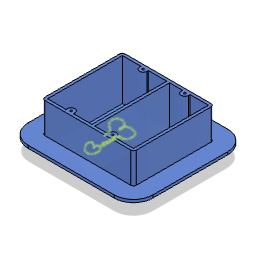
two-gang thicc (Autodesk Fusion 360 design; units mm, degrees)
Autodesk Fusion 360 part; units mm, degrees
note: some values were not read from the file. Set by a fixed rule: which sketch regions a step uses.
(part 1 of 2)
sketch "bottom" plane through (0, 0, 0) normal (0, 1, 0) x (1, 0, 0)
  line L0 (3.175, 0) -> (101.6, 0)
  line L1 (104.775, 3.175) -> (104.775, 88.9)
  line L2 (101.6, 92.075) -> (3.175, 92.075)
  line L3 (0, 88.9) -> (0, 3.175)
  arc A0 (0, 3.175) -> (3.175, 0) centre (3.175, 3.175) ccw
  arc A1 (101.6, 0) -> (104.775, 3.175) centre (101.6, 3.175) ccw
  arc A2 (3.175, 92.075) -> (0, 88.9) centre (3.175, 88.9) ccw
  arc A3 (104.775, 88.9) -> (101.6, 92.075) centre (101.6, 88.9) ccw
  point P0 (104.775, 0)
  point P1 (0, 92.075)
  dimension "d1" = 104.775
  dimension "d2" = 92.075
  dimension "d12" = 3.175
  dimension "d13" = 3.175
  dimension "d14" = 3.175
  dimension "d15" = 3.175
  constraint horizontal L0
  constraint vertical L1
  constraint horizontal L2
  constraint vertical L3
  constraint coincident origin L0
  constraint coincident origin L3
  constraint tangent L0 A0
  constraint tangent L3 A0
  constraint coincident P0 L0
  constraint coincident P0 L1
  constraint tangent L0 A1
  constraint tangent L1 A1
  constraint coincident P1 L2
  constraint coincident P1 L3
  constraint tangent L2 A2
  constraint tangent L3 A2
  constraint tangent L1 A3
  constraint tangent L2 A3
  measures "d1" distance of origin P0
  measures "d2" distance of origin P1
  measures "d12" radius of A0
  measures "d13" radius of A1
  measures "d14" radius of A2
  measures "d15" radius of A3
extrude "Extrude1" add sketch "bottom" along normal blind 50.8
sketch "top" plane through (0, 50.8, 0) normal (0, 1, 0) x (-1, 0, 0)
  line L0 (0, -88.9) -> (0, -3.175)
  line L1 (-3.175, 0) -> (-101.6, 0)
  line L2 (-104.775, -3.175) -> (-104.775, -88.9)
  line L3 (-101.6, -92.075) -> (-3.175, -92.075)
  line L4 (-3.175, -92.075) -> (-53.975, -92.075)
  line L5 (-57.15, -88.9) -> (-57.15, -3.175)
  line L6 (-53.975, 0) -> (-3.175, 0)
  line L7 (0, -3.175) -> (0, -88.9)
  arc A0 (-3.175, -92.075) -> (0, -88.9) centre (-3.175, -88.9) ccw
  arc A1 (-57.15, -88.9) -> (-53.975, -92.075) centre (-53.975, -88.9) ccw
  arc A2 (0, -3.175) -> (-3.175, 0) centre (-3.175, -3.175) ccw
  arc A3 (-53.975, 0) -> (-57.15, -3.175) centre (-53.975, -3.175) ccw
  line L8 (-3.175, -3.175) -> (-3.175, -88.9)
  line L9 (-53.975, -3.175) -> (-3.175, -3.175)
  line L10 (-53.975, -88.9) -> (-53.975, -3.175)
  line L11 (-3.175, -88.9) -> (-53.975, -88.9)
  line L12 (-28.575, -83.0404) -> (-28.575, -83.0404)
  line L13 (-32.8083, -87.2737) -> (-32.8083, -88.9)
  line L14 (-32.8083, -88.9) -> (-28.575, -88.9)
  line L15 (-28.575, -88.9) -> (-28.575, -83.0404)
  line L16 (-28.575, -88.9) -> (-28.575, -3.175)
  line L17 (-3.175, -46.0375) -> (-53.975, -46.0375)
  arc A4 (-28.575, -83.0404) -> (-32.8083, -87.2737) centre (-28.575, -87.2737) ccw
  arc A5 (-24.3417, -87.2737) -> (-28.575, -83.0404) centre (-28.575, -87.2737) ccw
  line L18 (-24.3417, -87.2737) -> (-24.3417, -88.9)
  arc A6 (-28.575, -9.0346) -> (-24.3417, -4.8013) centre (-28.575, -4.8013) ccw
  line L19 (-24.3417, -4.8013) -> (-24.3417, -3.175)
  line L20 (-32.8083, -4.8013) -> (-32.8083, -3.175)
  arc A7 (-32.8083, -4.8013) -> (-28.575, -9.0346) centre (-28.575, -4.8013) ccw
  arc A8 (-104.775, -88.9) -> (-101.6, -92.075) centre (-101.6, -88.9) ccw
  arc A9 (-3.175, -92.075) -> (0, -88.9) centre (-3.175, -88.9) ccw
  arc A10 (0, -3.175) -> (-3.175, 0) centre (-3.175, -3.175) ccw
  arc A11 (-101.6, 0) -> (-104.775, -3.175) centre (-101.6, -3.175) ccw
  line L21 (-3.175, 0) -> (-52.3875, 0)
  line L22 (-52.3875, 0) -> (-52.3875, -92.075)
  line L23 (-101.6, -3.175) -> (-101.6, -88.9)
  line L24 (-101.6, -88.9) -> (-50.8, -88.9)
  line L25 (-50.8, -3.175) -> (-101.6, -3.175)
  arc A12 (-80.4333, -4.8013) -> (-76.2, -9.0346) centre (-76.2, -4.8013) ccw
  arc A13 (-76.2, -9.0346) -> (-71.9667, -4.8013) centre (-76.2, -4.8013) ccw
  line L26 (-71.9667, -4.8013) -> (-71.9667, -3.175)
  line L27 (-80.4333, -4.8013) -> (-80.4333, -3.175)
  arc A14 (-76.2, -83.0404) -> (-80.4333, -87.2737) centre (-76.2, -87.2737) ccw
  arc A15 (-71.9667, -87.2737) -> (-76.2, -83.0404) centre (-76.2, -87.2737) ccw
  line L28 (-80.4333, -87.2737) -> (-80.4333, -88.9)
  line L29 (-71.9667, -87.2737) -> (-71.9667, -88.9)
  point P0 (-28.575, -88.9)
  point P1 (-28.575, -83.0404)
  point P2 (-28.575, -83.0404)
  point P3 (-28.575, -83.0404)
  point P4 (-32.8083, -83.0404)
  point P5 (0, 15.875)
  point P6 (0, -3.175)
  point P7 (0, -3.175)
  point P8 (0, -88.9)
  point P9 (-7.62, -3.175)
  point P10 (-7.62, 0)
  dimension "d5" = 3.175
  dimension "d6" = 3.175
  dimension "d7" = 3.175
  dimension "d8" = 3.175
  dimension "d9" = 3.175
  dimension "d10" = 4.2333
  dimension "d11" = 4.2333
  dimension "d43" = 49.2125
  constraint horizontal L4
  constraint vertical L5
  constraint horizontal L6
  constraint vertical L7
  constraint tangent L4 A0
  constraint tangent L7 A0
  constraint tangent L4 A1
  constraint tangent L5 A1
  constraint tangent L6 A2
  constraint tangent L7 A2
  constraint tangent L5 A3
  constraint tangent L6 A3
  constraint midpoint L11 P0
  constraint coincident P3 P2
  constraint vertical L13
  constraint horizontal L14
  constraint vertical L15
  constraint coincident P0 L14.end
  constraint midpoint L9 L16.end
  constraint perpendicular L9 L16
  constraint midpoint L8 L17.start
  constraint midpoint L10 L17.end
  constraint perpendicular L10 L17
  constraint coincident P4 L12
  constraint coincident P4 L13
  constraint tangent L13 A4
  constraint symmetric P3 L16 P2
  constraint symmetric L13.end L16 L18.end
  constraint symmetric L16 L13.start A5.start
  constraint symmetric L16 A4 A5
  constraint symmetric P3 L17 A6.start
  constraint symmetric L13.end L17 L20.end
  constraint symmetric L17 L13.start L20.start
  constraint symmetric L17 A4 A7
  constraint symmetric L17 P3 A6.start
  constraint symmetric L17 A5.start A6.end
  constraint symmetric L17 A5 A6
  constraint symmetric L17 L18.end L19.end
  constraint coincident L1.start L6.end
  constraint parallel L1 L21
  constraint midpoint L3 L22.end
  constraint symmetric A2.centre L22 A11.centre
  constraint symmetric A0.centre L22 A8.centre
  constraint symmetric A3.centre L22 L25.start
  constraint symmetric A1.centre L22 L24.end
  constraint symmetric P3 L22 A14.start
  constraint symmetric L13.end L22 L29.end
  constraint symmetric L13.start L22 A15.start
  constraint symmetric A4 L22 A15
  constraint symmetric A5.start L22 A14.end
  constraint symmetric A5 L22 A14
  constraint symmetric L18.end L22 L28.end
  constraint symmetric A6.end L22 A12.start
  constraint symmetric A6.start L22 A12.end
  constraint symmetric A6 L22 A12
  constraint symmetric L19.end L22 L27.end
  constraint symmetric L20.start L22 A13.end
  constraint symmetric L20.end L22 L26.end
  constraint symmetric A7 L22 A13
  measures "d5" radius of A0
  measures "d6" radius of A1
  measures "d7" radius of A2
  measures "d8" radius of A3
  measures "d10" distance of P3 P4
  measures "d11" radius of A4
  measures "d43" distance of L1.start L21.end
extrude "Extrude2" cut sketch "top" against normal blind 47.625 contours L11 L13 L16 L17 A4 L22 L24 | L10 L11 L17 L22 L24 | L9 L10 L17 L22 L25 | L9 L16 L17 L20 A7 L22 L25 | L8 L11 L16 L17 A5 L18 | L8 L9 L16 L17 A6 L19
sketch "Sketch4" plane through (3.175, 0, 0) normal (1, 0, 0) x (0, 0, -1)
  line L0 (88.9, 50.8) -> (3.175, 50.8)
  line L1 (3.175, 50.8) -> (3.175, 3.175)
  line L2 (3.175, 3.175) -> (88.9, 3.175)
  line L3 (88.9, 3.175) -> (88.9, 50.8)
  line L4 (0, 15.875) -> (-19.05, 15.875)
  line L5 (-19.05, 15.875) -> (-19.05, 12.7)
  line L6 (-19.05, 12.7) -> (0, 12.7)
  line L7 (0, 12.7) -> (0, 15.875)
  point P0 (0, 15.875)
  point P1 (-19.05, 12.7)
  constraint horizontal L4
  constraint vertical L5
  constraint horizontal L6
  constraint vertical L7
  constraint coincident P1 L5.end
  constraint coincident P0 L4.start
sweep "Sweep1" add profiles "Sketch4" along 8 edges at (103.8451, 50.8, -91.1451) (52.3875, 50.8, -92.075) (0.9299, 50.8, -91.1451) (0, 50.8, -46.0375) (0.9299, 50.8, -0.9299) (52.3875, 50.8, 0) (103.8451, 50.8, -0.9299) (104.775, 50.8, -46.0375) section 1 contours L4 L5 L6 L7
sketch "wire-cutouts" plane through (0, 0, 0) normal (0, 0, 1) x (1, 0, 0)
  line L0 (101.6, 12.7) -> (3.175, 12.7)
  line L1 (3.175, 12.7) -> (3.175, 0)
  line L2 (3.175, 0) -> (101.6, 0)
  line L3 (101.6, 0) -> (101.6, 12.7)
  line L4 (7.62, 0) -> (22.86, 0)
  line L5 (22.86, 0) -> (22.86, 10.16)
  line L6 (22.86, 10.16) -> (7.62, 10.16)
  line L7 (7.62, 10.16) -> (7.62, 0)
  line L8 (7.62, 0) -> (34.7663, 0)
  line L9 (34.7663, 0) -> (34.7663, 3.175)
  line L10 (34.7663, 3.175) -> (7.62, 3.175)
  line L11 (7.62, 3.175) -> (7.62, 0)
  line L12 (52.3875, 12.7) -> (52.3875, 0)
  line L13 (70.0087, 3.175) -> (97.155, 3.175)
  line L14 (81.915, 0) -> (81.915, 10.16)
  line L15 (97.155, 10.16) -> (97.155, 0)
  line L16 (81.915, 10.16) -> (97.155, 10.16)
  line L17 (3.175, 6.35) -> (7.62, 6.35)
  line L18 (22.86, 6.35) -> (81.915, 6.35)
  dimension "d27" = 15.24
  dimension "d28" = 10.16
  dimension "d29" = 3.175
  constraint horizontal L4
  constraint vertical L5
  constraint horizontal L6
  constraint vertical L7
  constraint coincident L2 L4.start
  constraint horizontal L8
  constraint vertical L9
  constraint horizontal L10
  constraint vertical L11
  constraint midpoint L0 L12.start
  constraint midpoint L2 L12.end
  constraint symmetric L4.start L12 L15.end
  constraint symmetric L4.end L12 L14.start
  constraint symmetric L5.end L12 L14.end
  constraint symmetric L6.end L12 L15.start
  constraint symmetric L9.end L12 L13.start
  constraint symmetric L10.end L12 L13.end
  constraint midpoint L1 L17.start
  constraint coincident L7 L17.end
  constraint perpendicular L7 L17
  constraint coincident L5 L18.start
  constraint coincident L14 L18.end
  constraint perpendicular L14 L18
  measures "d27" distance of L4.start L4.end
  measures "d28" distance of L4.start L6.end
  measures "d29" distance of L4.start L10.end
extrude "Extrude3" cut sketch "wire-cutouts" against normal blind 10.16 contours L5 L6 L7 L10 | L13 L14 L15 L16
sketch "top2" plane through (0, 50.8, 0) normal (0, 1, 0) x (-1, 0, 0)
  line L0 (-3.175, -88.9) -> (-24.3417, -88.9)
  line L1 (-24.3417, -88.9) -> (-24.3417, -87.2737)
  arc A0 (-24.3417, -87.2737) -> (-32.8083, -87.2737) centre (-28.575, -87.2737) ccw
  line L2 (-32.8083, -87.2737) -> (-32.8083, -88.9)
  line L3 (-32.8083, -88.9) -> (-53.975, -88.9)
  line L4 (-53.975, -88.9) -> (-53.975, -3.175)
  line L5 (-53.975, -3.175) -> (-32.8083, -3.175)
  line L6 (-32.8083, -3.175) -> (-32.8083, -4.8013)
  arc A1 (-32.8083, -4.8013) -> (-24.3417, -4.8013) centre (-28.575, -4.8013) ccw
  line L7 (-24.3417, -4.8013) -> (-24.3417, -3.175)
  line L8 (-24.3417, -3.175) -> (-3.175, -3.175)
  line L9 (-3.175, -3.175) -> (-3.175, -88.9)
  arc A2 (-104.775, -88.9) -> (-104.6625, -92.2792) centre (-53.975, -88.9) ccw
  line L10 (-101.6, -92.075) -> (-3.175, -92.075)
  arc A3 (-3.175, -92.075) -> (0, -88.9) centre (-3.175, -88.9) ccw
  line L11 (0, -88.9) -> (0, -3.175)
  arc A4 (0, -3.175) -> (-3.175, 0) centre (-3.175, -3.175) ccw
  line L12 (-3.175, 0) -> (-101.6, 0)
  arc A5 (-101.6, 0) -> (-101.7057, -3.175) centre (-53.975, -3.175) ccw
  line L13 (-104.775, -3.175) -> (-104.775, -88.9)
  circle A6 centre (-28.575, -4.8013) radius 4.2333 construction
  circle A7 centre (-28.575, -87.2737) radius 4.2333 construction
  circle A8 centre (-28.575, -87.2737) radius 1.27
  circle A9 centre (-28.575, -4.8013) radius 1.27
  line L14 (-52.3875, 0) -> (-52.3875, -92.075)
  circle A10 centre (-76.2, -4.8013) radius 1.27
  circle A11 centre (-76.2, -4.8013) radius 4.2333 construction
  circle A12 centre (-76.2, -87.2737) radius 4.2333 construction
  circle A13 centre (-76.2, -87.2737) radius 1.27
  point P0 (-101.6, -88.9)
  point P1 (-101.6, -3.175)
  point P2 (-101.6, -88.9)
  point P3 (-101.6, -3.175)
  dimension "d33" = 2.54
  dimension "d34" = 2.54
  constraint coincident L6.end A6
  constraint tangent L6 A6
  constraint coincident A1.end A6
  constraint coincident A0.end A7
  constraint tangent L2 A7
  constraint coincident L1.end A7
  constraint concentric A0 A8
  constraint concentric A6 A9
  constraint symmetric A6 L14 A11
  constraint symmetric A7 L14 A12
  constraint symmetric A8 L14 A13
  constraint symmetric A9 L14 A10
  measures "d33" diameter of A8
  measures "d34" diameter of A9
sketch "signature-bottom" plane through (0, 0, 0) normal (0, -1, 0) x (1, 0, 0)
  arc A0 (101.6, -92.075) -> (104.775, -88.9) centre (101.6, -88.9) ccw
  line L0 (104.775, -88.9) -> (104.775, -3.175)
  arc A1 (104.775, -3.175) -> (101.6, 0) centre (101.6, -3.175) ccw
  line L1 (101.6, 0) -> (3.175, 0)
  arc A2 (3.175, 0) -> (0, -3.175) centre (3.175, -3.175) ccw
  line L2 (0, -3.175) -> (0, -88.9)
  arc A3 (0, -88.9) -> (3.175, -92.075) centre (3.175, -88.9) ccw
  line L3 (3.175, -92.075) -> (101.6, -92.075)
  spline S0 degree 3 poles (12.8358, -24.6071) (12.9225, -26.3723) (13.5203, -28.1246) (14.5896, -29.7463) knots 0 0 0 0 1 1 1 1
  spline S1 degree 3 poles (14.5896, -29.7463) (15.5552, -31.209) (16.9043, -32.5055) (18.9989, -33.9781) knots 0 0 0 0 1 1 1 1
  spline S2 degree 3 poles (18.9989, -33.9781) (20.5126, -35.0431) (21.3902, -35.7105) (21.7552, -36.0741) knots 0 0 0 0 1 1 1 1
  spline S3 degree 3 poles (21.7552, -36.0741) (22.6967, -37.0156) (23.3286, -38.5421) (23.8413, -41.111) knots 0 0 0 0 1 1 1 1
  spline S4 degree 3 poles (23.8413, -41.111) (23.9364, -41.5924) (24.0301, -42.1306) (24.1608, -42.9599) knots 0 0 0 0 1 1 1 1
  spline S5 degree 3 poles (24.1608, -42.9599) (24.4107, -44.5418) (24.5271, -44.9764) (24.7032, -44.9764) knots 0 0 0 0 1 1 1 1
  spline S6 degree 3 poles (24.7032, -44.9764) (24.8665, -44.9764) (24.9006, -44.7478) (24.8878, -43.7551) knots 0 0 0 0 1 1 1 1
  spline S7 degree 3 poles (24.8878, -43.7551) (24.8793, -43.1332) (24.8694, -42.913) (24.8211, -42.2286) knots 0 0 0 0 1 1 1 1
  spline S8 degree 3 poles (24.8211, -42.2286) (24.7302, -40.9662) (24.6052, -40.0687) (24.3866, -39.1116) knots 0 0 0 0 1 1 1 1
  spline S9 degree 3 poles (24.3866, -39.1116) (24.0358, -37.5893) (23.5175, -36.3907) (22.9253, -35.7361) knots 0 0 0 0 1 1 1 1
  spline S10 degree 3 poles (22.9253, -35.7361) (22.6072, -35.3839) (21.6501, -34.6512) (20.4899, -33.8673) knots 0 0 0 0 1 1 1 1
  spline S11 degree 3 poles (20.4899, -33.8673) (19.858, -33.4399) (19.5058, -33.1914) (19.1338, -32.913) knots 0 0 0 0 1 1 1 1
  spline S12 degree 3 poles (19.1338, -32.913) (17.7038, -31.8381) (16.6828, -30.8114) (15.9174, -29.6753) knots 0 0 0 0 1 1 1 1
  spline S13 degree 3 poles (15.9174, -29.6753) (15.0298, -28.3561) (14.4575, -26.9943) (14.2346, -25.6708) knots 0 0 0 0 1 1 1 1
  spline S14 degree 3 poles (14.2346, -25.6708) (14.0585, -24.6185) (14.111, -23.6358) (14.3936, -22.7597) knots 0 0 0 0 1 1 1 1
  spline S15 degree 3 poles (14.3936, -22.7597) (14.6137, -22.078) (14.9588, -21.5057) (15.4402, -21.0272) knots 0 0 0 0 1 1 1 1
  spline S16 degree 3 poles (15.4402, -21.0272) (15.6575, -20.8099) (15.8009, -20.6935) (16.0452, -20.5302) knots 0 0 0 0 1 1 1 1
  spline S17 degree 3 poles (16.0452, -20.5302) (16.6558, -20.124) (17.3303, -19.8883) (18.1681, -19.7903) knots 0 0 0 0 1 1 1 1
  spline S18 degree 3 poles (18.1681, -19.7903) (18.4734, -19.7534) (19.1963, -19.7534) (19.4746, -19.7889) knots 0 0 0 0 1 1 1 1
  spline S19 degree 3 poles (19.4746, -19.7889) (21.0565, -19.9934) (22.8884, -20.8909) (24.4561, -22.2314) knots 0 0 0 0 1 1 1 1
  spline S20 degree 3 poles (24.4561, -22.2314) (24.6933, -22.433) (25.1775, -22.9059) (25.3749, -23.1289) knots 0 0 0 0 1 1 1 1
  spline S21 degree 3 poles (25.3749, -23.1289) (25.8535, -23.6685) (26.2241, -24.228) (26.4314, -24.7236) knots 0 0 0 0 1 1 1 1
  line L4 (26.4314, -24.7236) -> (26.4698, -24.8131)
  line L5 (26.4698, -24.8131) -> (26.3562, -25.0431)
  spline S22 degree 3 poles (26.3562, -25.0431) (26.2312, -25.2959) (26.1659, -25.4634) (26.0906, -25.7247) knots 0 0 0 0 1 1 1 1
  spline S23 degree 3 poles (26.0906, -25.7247) (25.8606, -26.5256) (25.8066, -27.6361) (25.9657, -28.3461) knots 0 0 0 0 1 1 1 1
  spline S24 degree 3 poles (25.9657, -28.3461) (26.0168, -28.5748) (26.0849, -28.7608) (26.2113, -29.0221) knots 0 0 0 0 1 1 1 1
  spline S25 degree 3 poles (26.2113, -29.0221) (26.4641, -29.5418) (26.8305, -30.0743) (27.0705, -30.2661) knots 0 0 0 0 1 1 1 1
  spline S26 degree 3 poles (27.0705, -30.2661) (27.177, -30.3527) (27.2877, -30.3853) (27.4439, -30.3754) knots 0 0 0 0 1 1 1 1
  spline S27 degree 3 poles (27.4439, -30.3754) (27.6484, -30.3626) (27.806, -30.2419) (27.9338, -30.0005) knots 0 0 0 0 1 1 1 1
  spline S28 degree 3 poles (27.9338, -30.0005) (28.0986, -29.6867) (28.1795, -29.2876) (28.1966, -28.7026) knots 0 0 0 0 1 1 1 1
  spline S29 degree 3 poles (28.1966, -28.7026) (28.2122, -28.1544) (28.144, -27.5083) (28.0077, -26.892) knots 0 0 0 0 1 1 1 1
  spline S30 degree 3 poles (28.0077, -26.892) (27.9111, -26.4561) (27.647, -25.4137) (27.576, -25.1837) knots 0 0 0 0 1 1 1 1
  spline S31 degree 3 poles (27.576, -25.1837) (27.4908, -24.9082) (27.4794, -24.9494) (27.6953, -24.7335) knots 0 0 0 0 1 1 1 1
  spline S32 degree 3 poles (27.6953, -24.7335) (28.1341, -24.2962) (28.8342, -23.9099) (29.9375, -23.4995) knots 0 0 0 0 1 1 1 1
  spline S33 degree 3 poles (29.9375, -23.4995) (30.5226, -23.2822) (30.7086, -23.2297) (31.0977, -23.1729) knots 0 0 0 0 1 1 1 1
  spline S34 degree 3 poles (31.0977, -23.1729) (32.15, -23.0195) (33.9407, -23.0664) (35.2301, -23.2794) knots 0 0 0 0 1 1 1 1
  spline S35 degree 3 poles (35.2301, -23.2794) (35.6959, -23.3561) (35.9444, -23.4186) (36.359, -23.5648) knots 0 0 0 0 1 1 1 1
  spline S36 degree 3 poles (36.359, -23.5648) (38.2235, -24.2209) (39.9177, -25.3768) (40.6689, -26.5058) knots 0 0 0 0 1 1 1 1
  spline S37 degree 3 poles (40.6689, -26.5058) (41.1006, -27.1547) (41.4741, -28.3845) (41.6232, -29.654) knots 0 0 0 0 1 1 1 1
  spline S38 degree 3 poles (41.6232, -29.654) (41.6516, -29.8997) (41.6558, -29.9977) (41.6558, -30.5202) knots 0 0 0 0 1 1 1 1
  spline S39 degree 3 poles (41.6558, -30.5202) (41.6558, -31.1195) (41.6487, -31.2402) (41.5905, -31.7131) knots 0 0 0 0 1 1 1 1
  spline S40 degree 3 poles (41.5905, -31.7131) (41.342, -33.721) (40.4502, -35.2788) (39.0713, -36.1167) knots 0 0 0 0 1 1 1 1
  spline S41 degree 3 poles (39.0713, -36.1167) (38.8683, -36.2402) (38.3613, -36.4887) (38.1653, -36.5612) knots 0 0 0 0 1 1 1 1
  spline S42 degree 3 poles (38.1653, -36.5612) (37.8487, -36.679) (37.6314, -36.7188) (37.1571, -36.7429) knots 0 0 0 0 1 1 1 1
  spline S43 degree 3 poles (37.1571, -36.7429) (36.6317, -36.7699) (36.2937, -36.7372) (35.3678, -36.5711) knots 0 0 0 0 1 1 1 1
  spline S44 degree 3 poles (35.3678, -36.5711) (34.53, -36.4191) (34.2062, -36.3879) (33.9151, -36.4291) knots 0 0 0 0 1 1 1 1
  spline S45 degree 3 poles (33.9151, -36.4291) (33.6851, -36.4603) (33.5658, -36.5299) (33.3258, -36.7685) knots 0 0 0 0 1 1 1 1
  spline S46 degree 3 poles (33.3258, -36.7685) (33.1227, -36.9701) (33.0716, -37.0596) (33.0716, -37.2101) knots 0 0 0 0 1 1 1 1
  spline S47 degree 3 poles (33.0716, -37.2101) (33.0716, -37.443) (33.2647, -37.8406) (33.5757, -38.2453) knots 0 0 0 0 1 1 1 1
  spline S48 degree 3 poles (33.5757, -38.2453) (33.6268, -38.3121) (33.668, -38.3703) (33.668, -38.376) knots 0 0 0 0 1 1 1 1
  spline S49 degree 3 poles (33.668, -38.376) (33.668, -38.4001) (33.5487, -38.4456) (33.4309, -38.4654) knots 0 0 0 0 1 1 1 1
  spline S50 degree 3 poles (33.4309, -38.4654) (33.3599, -38.4782) (33.1412, -38.4924) (32.9225, -38.5009) knots 0 0 0 0 1 1 1 1
  spline S51 degree 3 poles (32.9225, -38.5009) (32.4226, -38.518) (32.2252, -38.5535) (31.9881, -38.6728) knots 0 0 0 0 1 1 1 1
  spline S52 degree 3 poles (31.9881, -38.6728) (31.6799, -38.8276) (31.4272, -39.1272) (31.2766, -39.5163) knots 0 0 0 0 1 1 1 1
  spline S53 degree 3 poles (31.2766, -39.5163) (31.2028, -39.7094) (31.1787, -39.8415) (31.1787, -40.063) knots 0 0 0 0 1 1 1 1
  spline S54 degree 3 poles (31.1787, -40.063) (31.1801, -40.2902) (31.2099, -40.4564) (31.2965, -40.7091) knots 0 0 0 0 1 1 1 1
  spline S55 degree 3 poles (31.2965, -40.7091) (31.3832, -40.9562) (31.4485, -41.0769) (31.6061, -41.2686) knots 0 0 0 0 1 1 1 1
  spline S56 degree 3 poles (31.6061, -41.2686) (31.6473, -41.3183) (31.6757, -41.3638) (31.67, -41.3695) knots 0 0 0 0 1 1 1 1
  spline S57 degree 3 poles (31.67, -41.3695) (31.6643, -41.3751) (31.599, -41.4192) (31.5266, -41.4689) knots 0 0 0 0 1 1 1 1
  spline S58 degree 3 poles (31.5266, -41.4689) (31.0381, -41.7997) (31.0807, -42.2896) (31.6459, -42.8321) knots 0 0 0 0 1 1 1 1
  spline S59 degree 3 poles (31.6459, -42.8321) (31.8731, -43.0508) (32.123, -43.2382) (32.5533, -43.5152) knots 0 0 0 0 1 1 1 1
  spline S60 degree 3 poles (32.5533, -43.5152) (32.8614, -43.7111) (32.9836, -43.8063) (33.1426, -43.9681) knots 0 0 0 0 1 1 1 1
  spline S61 degree 3 poles (33.1426, -43.9681) (33.286, -44.113) (33.3528, -44.211) (33.3982, -44.3416) knots 0 0 0 0 1 1 1 1
  spline S62 degree 3 poles (33.3982, -44.3416) (33.4763, -44.5646) (33.3783, -44.762) (33.127, -44.8812) knots 0 0 0 0 1 1 1 1
  spline S63 degree 3 poles (33.127, -44.8812) (32.8969, -44.992) (32.7265, -45.0176) (32.1628, -45.0332) knots 0 0 0 0 1 1 1 1
  spline S64 degree 3 poles (32.1628, -45.0332) (31.9072, -45.0403) (31.6899, -45.0531) (31.6558, -45.0616) knots 0 0 0 0 1 1 1 1
  spline S65 degree 3 poles (31.6558, -45.0616) (31.5379, -45.0957) (31.4953, -45.188) (31.4953, -45.4081) knots 0 0 0 0 1 1 1 1
  spline S66 degree 3 poles (31.4953, -45.4081) (31.4953, -45.6396) (31.5422, -45.773) (31.6615, -45.8866) knots 0 0 0 0 1 1 1 1
  spline S67 degree 3 poles (31.6615, -45.8866) (31.7538, -45.9747) (31.8532, -46.0414) (32.1486, -46.2062) knots 0 0 0 0 1 1 1 1
  spline S68 degree 3 poles (32.1486, -46.2062) (32.4084, -46.351) (32.7052, -46.5384) (32.8515, -46.6492) knots 0 0 0 0 1 1 1 1
  spline S69 degree 3 poles (32.8515, -46.6492) (32.9907, -46.7557) (33.2207, -46.9886) (33.296, -47.0979) knots 0 0 0 0 1 1 1 1
  spline S70 degree 3 poles (33.296, -47.0979) (33.4493, -47.3195) (33.4905, -47.4459) (33.4905, -47.6887) knots 0 0 0 0 1 1 1 1
  spline S71 degree 3 poles (33.4905, -47.6887) (33.4891, -47.8179) (33.482, -47.8889) (33.4635, -47.9514) knots 0 0 0 0 1 1 1 1
  spline S72 degree 3 poles (33.4635, -47.9514) (33.3613, -48.2936) (33.1085, -48.4626) (32.5462, -48.5691) knots 0 0 0 0 1 1 1 1
  spline S73 degree 3 poles (32.5462, -48.5691) (32.2139, -48.6316) (31.998, -48.7168) (31.8589, -48.8418) knots 0 0 0 0 1 1 1 1
  spline S74 degree 3 poles (31.8589, -48.8418) (31.6487, -49.0292) (31.6558, -49.2905) (31.8773, -49.495) knots 0 0 0 0 1 1 1 1
  spline S75 degree 3 poles (31.8773, -49.495) (32.0435, -49.6498) (32.3204, -49.8315) (32.7805, -50.0886) knots 0 0 0 0 1 1 1 1
  spline S76 degree 3 poles (32.7805, -50.0886) (33.1568, -50.2987) (33.3414, -50.418) (33.4621, -50.5302) knots 0 0 0 0 1 1 1 1
  spline S77 degree 3 poles (33.4621, -50.5302) (33.6112, -50.6708) (33.6155, -50.7446) (33.4777, -50.8071) knots 0 0 0 0 1 1 1 1
  spline S78 degree 3 poles (33.4777, -50.8071) (33.3556, -50.8625) (33.1639, -50.8838) (32.6314, -50.898) knots 0 0 0 0 1 1 1 1
  spline S79 degree 3 poles (32.6314, -50.898) (32.3616, -50.9051) (32.0875, -50.9179) (32.0208, -50.9264) knots 0 0 0 0 1 1 1 1
  spline S80 degree 3 poles (32.0208, -50.9264) (31.5578, -50.9861) (31.3462, -51.094) (31.3278, -51.28) knots 0 0 0 0 1 1 1 1
  spline S81 degree 3 poles (31.3278, -51.28) (31.3093, -51.4717) (31.4854, -51.7074) (31.9072, -52.0625) knots 0 0 0 0 1 1 1 1
  spline S82 degree 3 poles (31.9072, -52.0625) (32.576, -52.6248) (33.3158, -53.5322) (33.6481, -54.1996) knots 0 0 0 0 1 1 1 1
  spline S83 degree 3 poles (33.6481, -54.1996) (33.783, -54.4737) (33.8157, -54.593) (33.8072, -54.8017) knots 0 0 0 0 1 1 1 1
  spline S84 degree 3 poles (33.8072, -54.8017) (33.8029, -54.9111) (33.7916, -54.9736) (33.7688, -55.0318) knots 0 0 0 0 1 1 1 1
  spline S85 degree 3 poles (33.7688, -55.0318) (33.678, -55.2661) (33.4195, -55.3911) (33.1753, -55.3172) knots 0 0 0 0 1 1 1 1
  spline S86 degree 3 poles (33.1753, -55.3172) (32.8799, -55.2263) (32.4993, -54.833) (32.2721, -54.3842) knots 0 0 0 0 1 1 1 1
  spline S87 degree 3 poles (32.2721, -54.3842) (32.1912, -54.2238) (32.1628, -54.1513) (32.0761, -53.8872) knots 0 0 0 0 1 1 1 1
  spline S88 degree 3 poles (32.0761, -53.8872) (31.9441, -53.4839) (31.8077, -53.2099) (31.6785, -53.0934) knots 0 0 0 0 1 1 1 1
  spline S89 degree 3 poles (31.6785, -53.0934) (31.5649, -52.9912) (31.4442, -52.9386) (31.305, -52.9315) knots 0 0 0 0 1 1 1 1
  spline S90 degree 3 poles (31.305, -52.9315) (31.1176, -52.9216) (31.0267, -52.9841) (31.0267, -53.1232) knots 0 0 0 0 1 1 1 1
  spline S91 degree 3 poles (31.0267, -53.1232) (31.0267, -53.4243) (31.6657, -55.0588) (31.9938, -55.5941) knots 0 0 0 0 1 1 1 1
  spline S92 degree 3 poles (31.9938, -55.5941) (32.2068, -55.9435) (32.522, -56.2388) (32.8486, -56.3993) knots 0 0 0 0 1 1 1 1
  spline S93 degree 3 poles (32.8486, -56.3993) (33.3911, -56.6648) (33.9648, -56.5953) (34.3738, -56.2175) knots 0 0 0 0 1 1 1 1
  spline S94 degree 3 poles (34.3738, -56.2175) (34.7174, -55.898) (34.8509, -55.4805) (34.8055, -54.86) knots 0 0 0 0 1 1 1 1
  spline S95 degree 3 poles (34.8055, -54.86) (34.77, -54.3672) (34.6677, -54.0051) (34.4405, -53.5677) knots 0 0 0 0 1 1 1 1
  spline S96 degree 3 poles (34.4405, -53.5677) (34.2545, -53.2099) (34.0287, -52.8989) (33.5473, -52.3323) knots 0 0 0 0 1 1 1 1
  spline S97 degree 3 poles (33.5473, -52.3323) (33.1866, -51.9077) (33.1227, -51.8267) (33.1341, -51.8097) knots 0 0 0 0 1 1 1 1
  spline S98 degree 3 poles (33.1341, -51.8097) (33.1383, -51.8026) (33.198, -51.7912) (33.2661, -51.787) knots 0 0 0 0 1 1 1 1
  spline S99 degree 3 poles (33.2661, -51.787) (33.7603, -51.7472) (34.0614, -51.6407) (34.2801, -51.4234) knots 0 0 0 0 1 1 1 1
  spline S100 degree 3 poles (34.2801, -51.4234) (34.4519, -51.2544) (34.5257, -51.0798) (34.5243, -50.8412) knots 0 0 0 0 1 1 1 1
  spline S101 degree 3 poles (34.5243, -50.8412) (34.5243, -50.6197) (34.4519, -50.4081) (34.3014, -50.1823) knots 0 0 0 0 1 1 1 1
  spline S102 degree 3 poles (34.3014, -50.1823) (34.1949, -50.0247) (34.0784, -49.8997) (33.7944, -49.6469) knots 0 0 0 0 1 1 1 1
  line L6 (33.7944, -49.6469) -> (33.5516, -49.4297)
  line L7 (33.5516, -49.4297) -> (33.7845, -49.2025)
  spline S103 degree 3 poles (33.7845, -49.2025) (34.0287, -48.9625) (34.1295, -48.8361) (34.2247, -48.6472) knots 0 0 0 0 1 1 1 1
  spline S104 degree 3 poles (34.2247, -48.6472) (34.3653, -48.3717) (34.4135, -48.1303) (34.4022, -47.7824) knots 0 0 0 0 1 1 1 1
  spline S105 degree 3 poles (34.4022, -47.7824) (34.3908, -47.4714) (34.3383, -47.2499) (34.2005, -46.9574) knots 0 0 0 0 1 1 1 1
  spline S106 degree 3 poles (34.2005, -46.9574) (34.0827, -46.7046) (33.9506, -46.5143) (33.6567, -46.1763) knots 0 0 0 0 1 1 1 1
  spline S107 degree 3 poles (33.6567, -46.1763) (33.465, -45.9562) (33.4337, -45.9108) (33.4536, -45.8739) knots 0 0 0 0 1 1 1 1
  spline S108 degree 3 poles (33.4536, -45.8739) (33.4607, -45.8597) (33.5644, -45.7588) (33.6822, -45.6523) knots 0 0 0 0 1 1 1 1
  spline S109 degree 3 poles (33.6822, -45.6523) (34.0713, -45.2973) (34.246, -45.0516) (34.3383, -44.7265) knots 0 0 0 0 1 1 1 1
  spline S110 degree 3 poles (34.3383, -44.7265) (34.378, -44.5816) (34.3809, -44.3217) (34.344, -44.1812) knots 0 0 0 0 1 1 1 1
  spline S111 degree 3 poles (34.344, -44.1812) (34.3085, -44.0463) (34.2062, -43.8446) (34.1082, -43.7154) knots 0 0 0 0 1 1 1 1
  spline S112 degree 3 poles (34.1082, -43.7154) (33.9506, -43.5066) (33.6652, -43.2652) (33.3655, -43.0891) knots 0 0 0 0 1 1 1 1
  spline S113 degree 3 poles (33.3655, -43.0891) (33.2974, -43.0494) (33.1866, -42.9841) (33.117, -42.9443) knots 0 0 0 0 1 1 1 1
  spline S114 degree 3 poles (33.117, -42.9443) (32.7989, -42.7568) (32.4723, -42.4743) (32.3857, -42.3095) knots 0 0 0 0 1 1 1 1
  line L8 (32.3857, -42.3095) -> (32.3459, -42.2357)
  line L9 (32.3459, -42.2357) -> (32.3999, -42.2101)
  spline S115 degree 3 poles (32.3999, -42.2101) (32.4496, -42.1874) (32.5306, -42.186) (33.3556, -42.186) knots 0 0 0 0 1 1 1 1
  spline S116 degree 3 poles (33.3556, -42.186) (34.2318, -42.186) (34.2588, -42.1846) (34.3056, -42.1576) knots 0 0 0 0 1 1 1 1
  spline S117 degree 3 poles (34.3056, -42.1576) (34.3993, -42.1022) (34.4334, -42.0213) (34.4348, -41.8523) knots 0 0 0 0 1 1 1 1
  spline S118 degree 3 poles (34.4348, -41.8523) (34.4363, -41.5796) (34.2772, -41.4816) (33.6155, -41.3482) knots 0 0 0 0 1 1 1 1
  spline S119 degree 3 poles (33.6155, -41.3482) (33.1667, -41.2573) (32.9907, -41.2033) (32.7535, -41.0812) knots 0 0 0 0 1 1 1 1
  spline S120 degree 3 poles (32.7535, -41.0812) (32.4212, -40.9108) (32.2096, -40.6836) (32.1415, -40.4223) knots 0 0 0 0 1 1 1 1
  spline S121 degree 3 poles (32.1415, -40.4223) (32.069, -40.1468) (32.1912, -39.8599) (32.451, -39.6966) knots 0 0 0 0 1 1 1 1
  spline S122 degree 3 poles (32.451, -39.6966) (32.6087, -39.5972) (32.7791, -39.5418) (33.0432, -39.5021) knots 0 0 0 0 1 1 1 1
  spline S123 degree 3 poles (33.0432, -39.5021) (33.6765, -39.4069) (34.0174, -39.2777) (34.2375, -39.0462) knots 0 0 0 0 1 1 1 1
  spline S124 degree 3 poles (34.2375, -39.0462) (34.3823, -38.8929) (34.476, -38.6799) (34.4874, -38.4711) knots 0 0 0 0 1 1 1 1
  spline S125 degree 3 poles (34.4874, -38.4711) (34.4973, -38.3192) (34.4774, -38.2453) (34.3567, -37.9897) knots 0 0 0 0 1 1 1 1
  spline S126 degree 3 poles (34.3567, -37.9897) (34.3085, -37.8846) (34.2531, -37.754) (34.2375, -37.6986) knots 0 0 0 0 1 1 1 1
  spline S127 degree 3 poles (34.2375, -37.6986) (34.2091, -37.6063) (34.1934, -37.46) (34.2105, -37.443) knots 0 0 0 0 1 1 1 1
  spline S128 degree 3 poles (34.2105, -37.443) (34.2233, -37.4302) (34.6365, -37.541) (34.8694, -37.6177) knots 0 0 0 0 1 1 1 1
  spline S129 degree 3 poles (34.8694, -37.6177) (35.1364, -37.7071) (35.355, -37.7639) (35.6561, -37.8179) knots 0 0 0 0 1 1 1 1
  spline S130 degree 3 poles (35.6561, -37.8179) (36.4385, -37.9613) (36.9739, -37.9826) (37.6158, -37.896) knots 0 0 0 0 1 1 1 1
  spline S131 degree 3 poles (37.6158, -37.896) (38.0006, -37.8449) (38.4593, -37.7299) (38.837, -37.5907) knots 0 0 0 0 1 1 1 1
  spline S132 degree 3 poles (38.837, -37.5907) (39.1111, -37.4899) (39.5343, -37.2754) (39.76, -37.1263) knots 0 0 0 0 1 1 1 1
  spline S133 degree 3 poles (39.76, -37.1263) (40.2088, -36.8281) (40.6859, -36.3595) (41.085, -35.8241) knots 0 0 0 0 1 1 1 1
  spline S134 degree 3 poles (41.085, -35.8241) (41.6899, -35.0133) (42.1628, -34.0377) (42.4496, -33.0025) knots 0 0 0 0 1 1 1 1
  spline S135 degree 3 poles (42.4496, -33.0025) (42.6541, -32.2683) (42.7464, -31.439) (42.7464, -30.3427) knots 0 0 0 0 1 1 1 1
  spline S136 degree 3 poles (42.7464, -30.3427) (42.7464, -29.4197) (42.6811, -28.7821) (42.5291, -28.2297) knots 0 0 0 0 1 1 1 1
  spline S137 degree 3 poles (42.5291, -28.2297) (42.2948, -27.3762) (41.8347, -26.4348) (41.2568, -25.6282) knots 0 0 0 0 1 1 1 1
  spline S138 degree 3 poles (41.2568, -25.6282) (40.5894, -24.6938) (39.7998, -23.9383) (38.9691, -23.4399) knots 0 0 0 0 1 1 1 1
  spline S139 degree 3 poles (38.9691, -23.4399) (37.39, -22.4927) (34.1508, -21.7031) (32.2338, -21.7997) knots 0 0 0 0 1 1 1 1
  spline S140 degree 3 poles (32.2338, -21.7997) (31.048, -21.8593) (29.9659, -22.1419) (28.925, -22.6631) knots 0 0 0 0 1 1 1 1
  spline S141 degree 3 poles (28.925, -22.6631) (28.4493, -22.9002) (28.1014, -23.1203) (27.718, -23.4271) knots 0 0 0 0 1 1 1 1
  spline S142 degree 3 poles (27.718, -23.4271) (27.62, -23.5052) (27.4794, -23.6159) (27.4056, -23.6742) knots 0 0 0 0 1 1 1 1
  spline S143 degree 3 poles (27.4056, -23.6742) (27.3317, -23.7324) (27.2252, -23.8204) (27.1699, -23.8701) knots 0 0 0 0 1 1 1 1
  spline S144 degree 3 poles (27.1699, -23.8701) (27.1131, -23.9184) (27.0648, -23.9596) (27.0605, -23.9596) knots 0 0 0 0 1 1 1 1
  spline S145 degree 3 poles (27.0605, -23.9596) (27.0534, -23.9596) (26.43, -23.1445) (26.0494, -22.6404) knots 0 0 0 0 1 1 1 1
  spline S146 degree 3 poles (26.0494, -22.6404) (25.5524, -21.9772) (24.8523, -21.351) (23.9137, -20.7233) knots 0 0 0 0 1 1 1 1
  spline S147 degree 3 poles (23.9137, -20.7233) (22.3488, -19.6796) (20.5922, -18.9525) (19.2119, -18.7778) knots 0 0 0 0 1 1 1 1
  spline S148 degree 3 poles (19.2119, -18.7778) (17.282, -18.5322) (15.2798, -19.1385) (14.1693, -20.3058) knots 0 0 0 0 1 1 1 1
  spline S149 degree 3 poles (14.1693, -20.3058) (13.4181, -21.0968) (12.958, -22.2456) (12.8515, -23.6046) knots 0 0 0 0 1 1 1 1
  spline S150 degree 3 poles (12.8515, -23.6046) (12.8302, -23.8673) (12.8231, -24.3473) (12.8358, -24.6071) knots 0 0 0 0 1 1 1 1
  spline S151 degree 3 poles (26.768, -27.0255) (26.7864, -26.7969) (26.8177, -26.6108) (26.8802, -26.3751) knots 0 0 0 0 1 1 1 1
  spline S152 degree 3 poles (26.8802, -26.3751) (26.937, -26.1649) (26.9355, -26.1635) (27.0278, -26.4433) knots 0 0 0 0 1 1 1 1
  spline S153 degree 3 poles (27.0278, -26.4433) (27.2196, -27.0227) (27.3261, -27.7625) (27.3275, -28.5251) knots 0 0 0 0 1 1 1 1
  spline S154 degree 3 poles (27.3275, -28.5251) (27.3275, -28.8204) (27.3246, -28.873) (27.3019, -28.9213) knots 0 0 0 0 1 1 1 1
  spline S155 degree 3 poles (27.3019, -28.9213) (27.2792, -28.9724) (27.2764, -28.9752) (27.2522, -28.9539) knots 0 0 0 0 1 1 1 1
  spline S156 degree 3 poles (27.2522, -28.9539) (27.1841, -28.8929) (26.9938, -28.4583) (26.9043, -28.163) knots 0 0 0 0 1 1 1 1
  spline S157 degree 3 poles (26.9043, -28.163) (26.7666, -27.7085) (26.7339, -27.4402) (26.768, -27.0255) knots 0 0 0 0 1 1 1 1
  spline S158 degree 3 poles (22.1329, -61.9815) (22.2025, -62.8719) (22.3701, -63.562) (22.7407, -64.4964) knots 0 0 0 0 1 1 1 1
  spline S159 degree 3 poles (22.7407, -64.4964) (23.6808, -66.8594) (25.3905, -69.0591) (27.5192, -70.6396) knots 0 0 0 0 1 1 1 1
  spline S160 degree 3 poles (27.5192, -70.6396) (28.0205, -71.0116) (28.269, -71.165) (28.8611, -71.4689) knots 0 0 0 0 1 1 1 1
  spline S161 degree 3 poles (28.8611, -71.4689) (30.7257, -72.426) (32.3275, -72.737) (33.6893, -72.409) knots 0 0 0 0 1 1 1 1
  spline S162 degree 3 poles (33.6893, -72.409) (35.3792, -72.0028) (36.626, -70.6524) (37.3502, -68.4428) knots 0 0 0 0 1 1 1 1
  spline S163 degree 3 poles (37.3502, -68.4428) (37.6271, -67.5978) (37.7081, -67.0696) (37.7251, -65.979) knots 0 0 0 0 1 1 1 1
  spline S164 degree 3 poles (37.7251, -65.979) (37.7365, -65.276) (37.7052, -64.6867) (37.63, -64.1073) knots 0 0 0 0 1 1 1 1
  spline S165 degree 3 poles (37.63, -64.1073) (37.5533, -63.528) (37.4581, -63.1587) (37.2238, -62.5183) knots 0 0 0 0 1 1 1 1
  spline S166 degree 3 poles (37.2238, -62.5183) (36.7211, -61.1494) (36.0523, -60.1369) (34.9915, -59.1386) knots 0 0 0 0 1 1 1 1
  spline S167 degree 3 poles (34.9915, -59.1386) (34.2687, -58.4598) (33.7248, -58.0934) (33.2321, -57.9557) knots 0 0 0 0 1 1 1 1
  spline S168 degree 3 poles (33.2321, -57.9557) (32.8344, -57.8435) (32.4993, -57.7952) (32.106, -57.7952) knots 0 0 0 0 1 1 1 1
  spline S169 degree 3 poles (32.106, -57.7952) (31.7098, -57.7938) (31.4286, -57.835) (31.1048, -57.9429) knots 0 0 0 0 1 1 1 1
  spline S170 degree 3 poles (31.1048, -57.9429) (30.5595, -58.1247) (30.1193, -58.457) (29.8097, -58.9213) knots 0 0 0 0 1 1 1 1
  spline S171 degree 3 poles (29.8097, -58.9213) (29.5967, -59.2394) (29.4434, -59.6711) (29.3866, -60.1042) knots 0 0 0 0 1 1 1 1
  spline S172 degree 3 poles (29.3866, -60.1042) (29.3582, -60.3257) (29.3582, -60.7532) (29.388, -60.9506) knots 0 0 0 0 1 1 1 1
  spline S173 degree 3 poles (29.388, -60.9506) (29.5087, -61.777) (29.9816, -62.656) (30.4133, -62.8591) knots 0 0 0 0 1 1 1 1
  spline S174 degree 3 poles (30.4133, -62.8591) (30.4914, -62.896) (30.5141, -62.9003) (30.6035, -62.8946) knots 0 0 0 0 1 1 1 1
  spline S175 degree 3 poles (30.6035, -62.8946) (30.7342, -62.8875) (30.7626, -62.8591) (30.7541, -62.7413) knots 0 0 0 0 1 1 1 1
  spline S176 degree 3 poles (30.7541, -62.7413) (30.747, -62.6333) (30.6887, -62.5183) (30.5141, -62.257) knots 0 0 0 0 1 1 1 1
  spline S177 degree 3 poles (30.5141, -62.257) (30.3508, -62.017) (30.2713, -61.8466) (30.2102, -61.6123) knots 0 0 0 0 1 1 1 1
  spline S178 degree 3 poles (30.2102, -61.6123) (30.0327, -60.9264) (30.1619, -60.0574) (30.5311, -59.4496) knots 0 0 0 0 1 1 1 1
  spline S179 degree 3 poles (30.5311, -59.4496) (30.8308, -58.9611) (31.1772, -58.7566) (31.758, -58.7268) knots 0 0 0 0 1 1 1 1
  spline S180 degree 3 poles (31.758, -58.7268) (31.8518, -58.7225) (32.008, -58.7268) (32.106, -58.7353) knots 0 0 0 0 1 1 1 1
  spline S181 degree 3 poles (32.106, -58.7353) (32.9026, -58.8091) (33.5686, -59.1514) (34.3624, -59.8983) knots 0 0 0 0 1 1 1 1
  spline S182 degree 3 poles (34.3624, -59.8983) (35.4928, -60.9605) (36.2653, -62.4743) (36.5493, -64.1826) knots 0 0 0 0 1 1 1 1
  spline S183 degree 3 poles (36.5493, -64.1826) (36.643, -64.7464) (36.67, -65.1312) (36.6601, -65.7716) knots 0 0 0 0 1 1 1 1
  spline S184 degree 3 poles (36.6601, -65.7716) (36.6501, -66.3723) (36.6132, -66.7472) (36.5067, -67.2783) knots 0 0 0 0 1 1 1 1
  spline S185 degree 3 poles (36.5067, -67.2783) (36.3051, -68.2937) (35.9089, -69.2479) (35.3579, -70.0446) knots 0 0 0 0 1 1 1 1
  spline S186 degree 3 poles (35.3579, -70.0446) (34.9503, -70.6353) (34.1523, -71.1749) (33.269, -71.4575) knots 0 0 0 0 1 1 1 1
  spline S187 degree 3 poles (33.269, -71.4575) (32.9111, -71.5711) (32.6314, -71.6166) (32.2622, -71.6166) knots 0 0 0 0 1 1 1 1
  spline S188 degree 3 poles (32.2622, -71.6166) (31.9782, -71.6166) (31.7353, -71.591) (31.4371, -71.5314) knots 0 0 0 0 1 1 1 1
  spline S189 degree 3 poles (31.4371, -71.5314) (28.9918, -71.0386) (25.906, -68.4215) (24.1792, -65.3754) knots 0 0 0 0 1 1 1 1
  spline S190 degree 3 poles (24.1792, -65.3754) (23.2789, -63.7893) (22.8586, -62.2073) (23.0119, -60.9946) knots 0 0 0 0 1 1 1 1
  spline S191 degree 3 poles (23.0119, -60.9946) (23.1383, -60.0105) (23.624, -59.4013) (24.4135, -59.2408) knots 0 0 0 0 1 1 1 1
  spline S192 degree 3 poles (24.4135, -59.2408) (24.574, -59.2082) (24.8438, -59.1982) (25.027, -59.2181) knots 0 0 0 0 1 1 1 1
  spline S193 degree 3 poles (25.027, -59.2181) (25.649, -59.2863) (26.1346, -59.5305) (26.8092, -60.1198) knots 0 0 0 0 1 1 1 1
  spline S194 degree 3 poles (26.8092, -60.1198) (27.194, -60.4564) (27.3232, -60.5402) (27.4553, -60.5402) knots 0 0 0 0 1 1 1 1
  spline S195 degree 3 poles (27.4553, -60.5402) (27.5206, -60.5402) (27.5362, -60.5345) (27.5604, -60.5032) knots 0 0 0 0 1 1 1 1
  spline S196 degree 3 poles (27.5604, -60.5032) (27.6541, -60.384) (27.5447, -60.1823) (27.211, -59.8571) knots 0 0 0 0 1 1 1 1
  spline S197 degree 3 poles (27.211, -59.8571) (26.5323, -59.1968) (25.3919, -58.518) (24.7302, -58.3803) knots 0 0 0 0 1 1 1 1
  spline S198 degree 3 poles (24.7302, -58.3803) (24.547, -58.3419) (24.236, -58.3377) (24.0443, -58.3717) knots 0 0 0 0 1 1 1 1
  spline S199 degree 3 poles (24.0443, -58.3717) (23.4294, -58.4825) (22.8969, -58.8702) (22.6157, -59.4169) knots 0 0 0 0 1 1 1 1
  spline S200 degree 3 poles (22.6157, -59.4169) (22.3559, -59.9196) (22.1855, -60.5572) (22.1372, -61.2076) knots 0 0 0 0 1 1 1 1
  spline S201 degree 3 poles (22.1372, -61.2076) (22.1244, -61.3823) (22.1216, -61.8424) (22.1329, -61.9815) knots 0 0 0 0 1 1 1 1
extrude "Extrude4" add sketch "signature-bottom" along normal blind 0.762 contours S0 S1 S2 S3 S4 S5 S6 S7 S8 S9 S10 S11 S12 S13 S14 S15 S16 S17 S18 S19 S20 S21 L4 L5 S22 S23 S24 S25 S26 S27 S28 S29 S30 S31 S32 S33 S34 S35 S36 S37 S38 S39 S40 S41 S42 S43 S44 S45 S46 S47 S48 S49 S50 S51 S52 S53 S54 S55 S56 S57 S58 S59 S60 S61 S62 S63 S64 S65 S66 S67 S68 S69 S70 S71 S72 S73 S74 S75 S76 S77 S78 S79 S80 S81 S82 S83 S84 S85 S86 S87 S88 S89 S90 S91 S92 S93 S94 S95 S96 S97 S98 S99 S100 S101 S102 L6 L7 S103 S104 S105 S106 S107 S108 S109 S110 S111 S112 S113 S114 L8 L9 S115 S116 S117 S118 S119 S120 S121 S122 S123 S124 S125 S126 S127 S128 S129 S130 S131 S132 S133 S134 S135 S136 S137 S138 S139 S140 S141 S142 S143 S144 S145 S146 S147 S148 S149 S150 | S158 S159 S160 S161 S162 S163 S164 S165 S166 S167 S168 S169 S170 S171 S172 S173 S174 S175 S176 S177 S178 S179 S180 S181 S182 S183 S184 S185 S186 S187 S188 S189 S190 S191 S192 S193 S194 S195 S196 S197 S198 S199 S200 S201